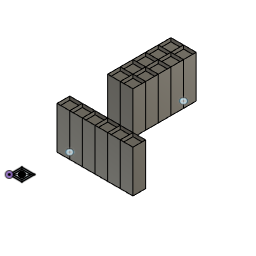
Standoffs (Autodesk Fusion 360 design; units mm, degrees)
Autodesk Fusion 360 part; units mm, degrees
sketch "Sketch1" plane through (0, 0, 0) normal (0, 0, 1) x (1, 0, 0)
  line L0 (0, 0) -> (2.5, 0)
  line L1 (2.5, 0) -> (2.5, 2.5)
  line L2 (2.5, 2.5) -> (0, 2.5)
  line L3 (0, 2.5) -> (0, 0)
  line L4 (2.5, 2.5) -> (0, 0) construction
  line L5 (0, 2.5) -> (2.5, 0) construction
  line L6 (0.35, 2.15) -> (2.15, 2.15)
  line L7 (2.15, 2.15) -> (2.15, 0.35)
  line L8 (2.15, 0.35) -> (0.35, 0.35)
  line L9 (0.35, 0.35) -> (0.35, 2.15)
  point P0 (1.25, 1.25)
  dimension "d22" = 2.5
  dimension "d23" = 2.5
  dimension "d24" = 1.8
  dimension "d25" = 1.8
  dimension "d26" = 0.35
  dimension "d27" = 0.35
  constraint horizontal L0
  constraint vertical L1
  constraint horizontal L2
  constraint vertical L3
  constraint coincident L0.start L3.end
  constraint midpoint L5 P0
  constraint horizontal L6
  constraint vertical L7
  constraint horizontal L8
  constraint vertical L9
  constraint coincident L5 L6.start
  measures "d22" distance of L0.start L0.end
  measures "d23" distance of L0.start L2.end
  measures "d24" distance of L6.start L6.end
  measures "d25" distance of L6.start L8.end
  measures "d26" distance of L2 L6
  measures "d27" distance of L0 L8
extrude "Extrude1" add sketch "Sketch1" along normal blind 8 contours L0 L1 L2 L3 | L6 L7 L8 L9 makes body 1
extrude "Extrude2" add sketch "Sketch1" along normal blind 0.35 from surface at 8 bodies 1
chamfer "Chamfer1" distance 0.35 angle 45 4 edges at (1.25, 2.15, 8.35) (2.15, 1.25, 8.35) (0.35, 1.25, 8.35) (1.25, 0.35, 8.35) on bodies 1
move_body "Move1" bodies 1 to x (1, 0, 0) y (0, 1, 0) z (0, 0, 1) at (-10.6424, 0, 0)
pattern_linear "R-Pattern1" count 5 spacing 2.5 along (1, 0, 0) count 2 spacing 2.5 along (0, 1, 0) of bodies 1 makes body 2 at (-8.1424, 1.6667, 2.7833) makes body 3 at (-4.8091, 0, 2.7833) makes body 4 at (-2.3091, 0, 2.7833) makes body 5 at (1.8576, 0.8333, 2.7833) makes body 6 at (-10.6424, 4.1667, 2.7833) makes body 7 at (-6.4757, 5, 2.7833) makes body 8 at (-3.9757, 5, 2.7833) makes body 9 at (-1.4757, 5, 2.7833) makes body 10 at (1.0243, 5, 2.7833)
copy_body "CopyPasteBodies1" bodies 1 makes body 11
move_body "Move2" bodies 11 to x (1, 0, 0) y (0, 1, 0) z (0, 0, 1) at (-6.7554, 0, 0)
pattern_linear "R-Pattern2" count 6 spacing 2.5 along (1, 0, 0) of bodies 11 makes body 12 at (-14.8978, 1.6667, 2.7833) makes body 13 at (-10.7311, 2.5, 2.7833) makes body 14 at (-8.2311, 2.5, 2.7833) makes body 15 at (-5.7311, 2.5, 2.7833) makes body 16 at (-3.2311, 2.5, 2.7833)
move_body "Move3" bodies 11 12 13 14 15 16 to x (1, 0, 0) y (0, 1, 0) z (0, 0, 1) at (19.8978, 6.95, 1.6)
move_body "Move4" bodies 6 7 8 9 10 5 4 3 2 1 to x (0, 1, 0) y (-1, 0, 0) z (0, 0, 1) at (-10.6424, 10.6424, 0)
move_body "Move5" bodies 6 7 8 9 10 5 4 3 2 1 to x (1, 0, 0) y (0, 1, 0) z (0, 0, 1) at (18.1424, 16.95, 1.6)
equation "d26 = d27"
